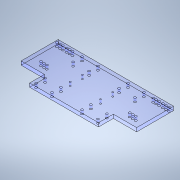
# Autodesk Inventor part: Plaque trans
Saved by Autodesk Inventor 2022 (Build 260153000, 153)
## iProperties
Created: 2022-04-30
Part Number: Plaque trans
Material: Générique
Document SubType Name: Modeling
Designer: victo
Density: 1 g/cm^3
Appearance: Transparent - Bleu
Author: victo
Autodesk Inventor part; units mm, degrees
ref_plane "YZ Plane" through (0, 0, 0) normal (1, 0, 0) x (0, 1, 0)
ref_plane "XZ Plane" through (0, 0, 0) normal (0, 1, 0) x (-1, 0, 0)
ref_plane "XY Plane" through (0, 0, 0) normal (0, 0, 1) x (1, 0, 0)
sketch "Esquisse1" plane through (0, 0, 0) normal (0, 1, 0) x (-1, 0, 0)
  line L0 (-75, -17.3205) -> (-55, -17.3205)
  line L1 (-55, -17.3205) -> (0, -17.3205)
  line L2 (0, -17.3205) -> (55, -17.3205)
  line L3 (55, -17.3205) -> (75, -17.3205)
  line L4 (75, -17.3205) -> (75, 17.3205)
  line L5 (75, 17.3205) -> (55, -17.3205)
  line L6 (-55, -17.3205) -> (-75, 17.3205)
  line L7 (-75, 17.3205) -> (-75, -17.3205)
  line L8 (-75, 25) -> (75, 25)
  line L9 (75, 25) -> (75, -25)
  line L10 (75, -25) -> (-75, -25)
  line L11 (-75, -25) -> (-75, 25)
  line L12 (-75, 17.3205) -> (-75, 25) construction
  line L13 (-75, -17.3205) -> (-75, -25) construction
  line L14 (75, 17.3205) -> (75, 25) construction
  line L15 (75, -17.3205) -> (75, -25) construction
  line L16 (-75, -25) -> (0, 0) construction
  line L17 (0, 0) -> (75, 25) construction
  line L18 (46.5, 45) -> (-46.5, 45)
  line L19 (-46.5, 45) -> (-46.5, 25)
  line L20 (-46.5, 25) -> (46.5, 25)
  line L21 (46.5, 25) -> (46.5, 45)
  line L22 (46.5, 45) -> (-46.5, 25) construction
  line L23 (-46.5, 45) -> (46.5, 25) construction
  line L24 (0, -39) -> (0, 59) projected
  line L25 (35, 25) -> (-35, 25)
  line L26 (-35, 25) -> (-35, 45)
  line L27 (-35, 45) -> (35, 45)
  line L28 (35, 45) -> (35, 25)
  line L29 (35, 25) -> (-35, 45) construction
  line L30 (-35, 25) -> (35, 45) construction
  line L31 (-41.75, 41) -> (-20.25, 41) construction
  line L32 (-20.25, 41) -> (-20.25, 29) construction
  line L33 (-20.25, 29) -> (-41.75, 29) construction
  line L34 (-41.75, 29) -> (-41.75, 41) construction
  line L35 (-41.75, 41) -> (-20.25, 29) construction
  line L36 (-20.25, 41) -> (-41.75, 29) construction
  line L37 (41.75, 29) -> (20.25, 29) construction
  line L38 (20.25, 29) -> (20.25, 41) construction
  line L39 (20.25, 41) -> (41.75, 41) construction
  line L40 (41.75, 41) -> (41.75, 29) construction
  line L41 (41.75, 29) -> (20.25, 41) construction
  line L42 (20.25, 29) -> (41.75, 41) construction
  circle A0 centre (-41.75, 41) radius 1.55
  circle A1 centre (-20.25, 41) radius 1.55
  circle A2 centre (-20.25, 29) radius 1.55
  circle A3 centre (-41.75, 29) radius 1.55
  circle A4 centre (20.25, 41) radius 1.55
  circle A5 centre (41.75, 41) radius 1.55
  circle A6 centre (41.75, 29) radius 1.55
  circle A7 centre (20.25, 29) radius 1.55
  line L43 (-44.5, 42.55) -> (-39, 42.55)
  line L44 (-39, 42.55) -> (-39, 39.45)
  line L45 (-39, 39.45) -> (-44.5, 39.45)
  line L46 (-44.5, 39.45) -> (-44.5, 42.55)
  line L47 (-44.5, 42.55) -> (-39, 39.45) construction
  line L48 (-39, 42.55) -> (-44.5, 39.45) construction
  line L49 (-31, 35) -> (0, 35)
  line L50 (0, 35) -> (31, 35)
  line L51 (0, 10) -> (12.5033, 10) construction
  circle A8 centre (-41.75, -21) radius 1.55
  circle A9 centre (-20.25, -21) radius 1.55
  circle A10 centre (-20.25, -9) radius 1.55
  circle A11 centre (-41.75, -9) radius 1.55
  circle A12 centre (20.25, -21) radius 1.55
  circle A13 centre (41.75, -21) radius 1.55
  circle A14 centre (41.75, -9) radius 1.55
  circle A15 centre (20.25, -9) radius 1.55
  line L52 (-31, -15) -> (0, -15)
  line L53 (0, -15) -> (31, -15)
  line L54 (-75, 17.3205) -> (-55, 17.3205)
  line L55 (-55, 17.3205) -> (-55, -17.3205)
  circle A16 centre (-60, 12.3205) radius 5
  circle A17 centre (-60, 12.3205) radius 1.55
  line L56 (-55, -17.3205) -> (-55, -25)
  line L57 (-75, -20.8205) -> (-55, -20.8205)
  circle A18 centre (-71.5, -20.8205) radius 3.5
  circle A19 centre (-58.5, -20.8205) radius 3.5
  line L58 (-71.5, -24.3205) -> (-58.5, -24.3205)
  circle A20 centre (-71.5, -20.8205) radius 1.55
  circle A21 centre (-58.5, -20.8205) radius 1.55
  circle A22 centre (60, 12.3205) radius 1.55
  circle A23 centre (71.5, -20.8205) radius 1.55
  circle A24 centre (58.5, -20.8205) radius 1.55
  circle A25 centre (-56, 12.3205) radius 1.55
  circle A26 centre (-67.5, -20.8205) radius 1.55
  circle A27 centre (-54.5, -20.8205) radius 1.55
  circle A28 centre (56, 12.3205) radius 1.55
  circle A29 centre (67.5, -20.8205) radius 1.55
  circle A30 centre (54.5, -20.8205) radius 1.55
  line L59 (-78, 25) -> (-75, 25)
  line L60 (-75, 25) -> (-75, -25)
  line L61 (-75, -25) -> (-78, -25)
  line L62 (-78, -25) -> (-78, 25)
  line L63 (-78, 25) -> (-75, -25) construction
  line L64 (-75, 25) -> (-78, -25) construction
  circle A31 centre (-64, 12.3205) radius 1.55
  circle A32 centre (-62.5, -20.8205) radius 1.55
  circle A33 centre (-75.5, -20.8205) radius 1.55
  circle A34 centre (64, 12.3205) radius 1.55
  circle A35 centre (62.5, -20.8205) radius 1.55
  circle A36 centre (75.5, -20.8205) radius 1.55
  line L65 (78, 25) -> (75, 25)
  line L66 (75, -25) -> (78, -25)
  line L67 (78, -25) -> (78, 25)
  line L68 (20.5, -0.25) -> (-20.5, -0.25) construction
  line L69 (-20.5, -0.25) -> (-20.5, 16.25) construction
  line L70 (-20.5, 16.25) -> (20.5, 16.25) construction
  line L71 (20.5, 16.25) -> (20.5, -0.25) construction
  line L72 (20.5, -0.25) -> (-20.5, 16.25) construction
  line L73 (-20.5, -0.25) -> (20.5, 16.25) construction
  circle A37 centre (-20.5, 16.25) radius 1.05
  circle A38 centre (20.5, 16.25) radius 1.05
  circle A39 centre (20.5, -0.25) radius 1.05
  circle A40 centre (-20.5, -0.25) radius 1.05
  point P0 (0, 0)
  point P1 (75, 17.3205)
  point P2 (46.5, 25)
  point P3 (-41.75, 39.45)
  point P4 (-41.75, 42.55)
  point P5 (-55, -22.2876)
  point P6 (-55, -19.3534)
  point P7 (-76.5, 0)
  point P8 (75, -22.2876)
  point P9 (75, -19.3534)
  point P10 (0, 8)
  dimension "d0" = 34.641
  dimension "d1" = 110
  dimension "d2" = 20
  dimension "d3" = 17.3205
  dimension "d4" = 60
  dimension "d6" = 50
  dimension "d7" = 70
  dimension "d8" = 93
  dimension "d10" = 11.5
  dimension "d11" = 11.5
  dimension "d12" = 12
  dimension "d13" = 21.5
  dimension "d14" = 3.1
  dimension "d15" = 5.5
  dimension "d16" = 4
  dimension "d20" = 50
  dimension "d23" = 10
  dimension "d24" = 3.1
  dimension "d25" = 7
  dimension "d26" = 3.1
  dimension "d27" = 2
  dimension "d28" = 70
  dimension "d29" = 150
  dimension "d32" = 4
  dimension "d39" = 4
  dimension "d44" = 3
  dimension "d47" = 4
  dimension "d54" = 4
  dimension "d59" = 41
  dimension "d60" = 16.5
  dimension "d61" = 8
  dimension "d62" = 2.1
  constraints: 146 end point, 41 centre point, 17 horizontal, 17 symmetric about line, 16 parallel, 15 coincident, 14 midpoint, 11 equal radius, 11 perpendicular, 11 point on line, 10 equal length, 8 tangent, 4 point on circle, 3 collinear, 1 vertical, 35 other
  measures "d0" distance of L12.start L7.end
  measures "d1" distance of L2.end L1.start
  measures "d2" distance of L7.end L1.start
  measures "d3" distance of L17.start L2.start
  measures "d4" angle of L6 L0
  measures "d6" distance between parallel lines of L10 L8
  measures "d7" distance between parallel lines of L10 L18
  measures "d8" distance between parallel lines of L21 L19
  measures "d10" distance between parallel lines of L19 L26
  measures "d11" distance between parallel lines of L21 L28
  measures "d12" distance of L33.end L31.start
  measures "d13" distance of L31.start L31.end
  measures "d14" diameter of A0
  measures "d15" distance between parallel lines of L46 L44
  measures "d16" distance between parallel lines of L26 L44
  measures "d20" distance between parallel lines of L52 L49
  measures "d23" diameter of A16
  measures "d24" diameter of A17
  measures "d25" distance between parallel lines of L58 L0
  measures "d26" diameter of A20
  measures "d27" distance between parallel lines of L19 L46
  measures "d28" distance between parallel lines of L28 L26
  measures "d29" distance between parallel lines of L4 L7
  measures "d32" distance of A17.centre A25.centre
  measures "d39" distance of A22.centre A28.centre
  measures "d44" distance between parallel lines of L62 L7
  measures "d47" distance of A17.centre A31.centre
  measures "d54" distance of A22.centre A34.centre
  measures "d59" distance of L69.end L70.end
  measures "d60" distance of L68.end L69.end
  measures "d61" distance of point (0, 8) L17.start
  measures "d62" diameter of A37
extrude "Extrusion1" add sketch "Esquisse1" against normal blind 5 contours L7 L6 L0 | L11 A33 L61 L62 L59 L7 | L0 A18 A33 L11 | L0 A19 A32 L57 A26 A18 | A18 A26 L57 A20 A33 | L54 A16 A31 A25 L55 L6 | L11 L8 L24 L1 L55 A25 L54 | L0 L56 A27 A19 | A19 A27 L57 A21 A32 | L1 L24 L10 L56 A27 | L54 L55 A25 A16 | A16 A25 A31 | A33 A18 L58 A19 A27 L56 L10 L11 | L57 A32 A19 L58 A18 A26 | A26 A18 A33 L57 A20 | L24 L8 L9 L5 L2 | L2 L3 L9 A36 L10 L24 | L19 L18 L26 L8 | A27 A19 A32 L57 A21 | L5 L4 L3 | L26 L18 L24 L8 | L4 L9 L65 L67 L66 A36 | L24 L18 L28 L8 | L28 L18 L21 L8 | A0 L43 L44 L45 | A0 L45 L46 L43
